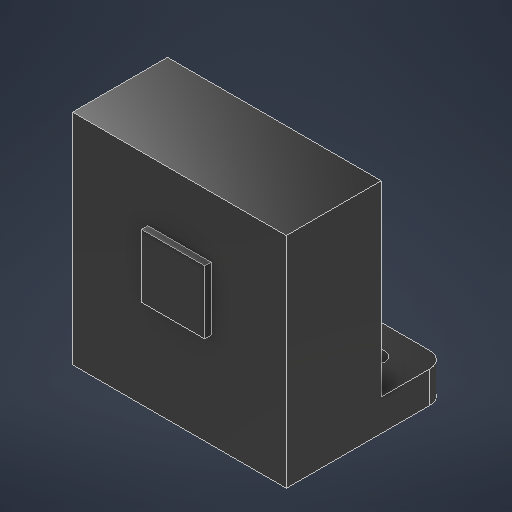
# Autodesk Inventor part: OGLiDAR
Saved by Autodesk Inventor 2027 (Build 310192060, 192F)
## iProperties
Created: 2026-07-12
Part Number: OGLiDAR
Material: LCP Plastic
Document SubType Name: Modeling
Designer: machnach0
Density: 1.626 g/cm^3
Appearance: Glossy - Black
Author: machnach0
Autodesk Inventor part; units mm, degrees
ref_plane "YZ Plane" through (0, 0, 0) normal (1, 0, 0) x (0, 1, 0)
ref_plane "XZ Plane" through (0, 0, 0) normal (0, 1, 0) x (-1, 0, 0)
ref_plane "XY Plane" through (0, 0, 0) normal (0, 0, 1) x (1, 0, 0)
sketch "Sketch1" plane through (0, 0, 0) normal (0, 0, 1) x (1, 0, 0)
  line L0 (0, 0) -> (42.926, 0)
  line L1 (42.926, 0) -> (42.926, 43.942)
  line L2 (42.926, 43.942) -> (0, 43.942)
  line L3 (0, 43.942) -> (0, 0)
  line L4 (0, 6.35) -> (42.926, 6.35)
  line L5 (15.113, 31.75) -> (27.813, 31.75)
  line L6 (27.813, 31.75) -> (27.813, 19.05)
  line L7 (27.813, 19.05) -> (15.113, 19.05)
  line L8 (15.113, 19.05) -> (15.113, 31.75)
  point P0 (21.463, 31.75)
  point P1 (21.463, 43.942)
  dimension "d0" = 43.942
  dimension "d1" = 42.926
  dimension "d2" = 12.7
  dimension "d3" = 6.35
  dimension "d4" = 12.7
  constraints: 18 end point, 4 parallel, 4 perpendicular, 2 horizontal, 2 midpoint, 2 point on line, 1 vertical alignment
  measures "d0" distance of L0.end L1.end
  measures "d1" distance of L1.end L2.end
  measures "d2" distance of L5.start L5.end
  measures "d3" distance between parallel lines of L0 L4
  measures "d4" distance between parallel lines of L4 L7
extrude "Extrusion1" add sketch "Sketch1" against normal blind 19.05 contours L3 L2 L1 L4 | L5 L6 L7 L8
extrude "Extrusion2" add sketch "Sketch1" against normal blind 32.004 contours L3 L4 L1 L0
extrude "Extrusion3" add sketch "Sketch1" along normal blind 1.27 contours L5 L6 L7 L8
sketch "Sketch2" plane through (0, 6.35, -19.05) normal (0, 1, 0) x (1, 0, 0)
  line L0 (0, 0) -> (0, 12.954) projected
  line L1 (42.926, 0) -> (42.926, 12.954) projected
  point P0 (0, -19.05)
  point P1 (35.306, 6.477)
  point P2 (7.62, 6.477)
  point P3 (0, 6.477)
  dimension "d11" = 7.62
  dimension "d12" = 7.62
  constraints: 2 horizontal alignment, 1 midpoint
  measures "d11" distance from line of L0 point (7.62, 6.477)
  measures "d12" distance from line of point (35.306, 6.477) L1
hole "Hole1" at (35.306, 6.35, -25.527) at (7.62, 6.35, -25.527) direction (0, -1, 0) diameter 3.81 end through all
fillet "Fillet1" radius 3.175 2 edges at (42.926, 3.175, -32.004) (0, 3.175, -32.004)
body "Solid1"
